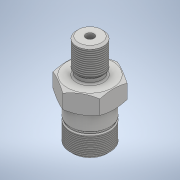
# Autodesk Inventor part: штрундель
Saved by Autodesk Inventor 2021 (Build 250183000, 183)
## iProperties
Created: 2020-04-22
Part Number: штрундель
Material: Типовые
Document SubType Name: Modeling
Designer: 2000
Density: 1 g/cm^3
Appearance: По умолчанию
Mass: 78.5301 g
Surface Area: 176.87 cm^2
Volume: 78.5301 cm^3
Author: 2000
Autodesk Inventor part; units mm, degrees
ref_plane "YZ Plane" through (0, 0, 0) normal (1, 0, 0) x (0, 1, 0)
ref_plane "XZ Plane" through (0, 0, 0) normal (0, 1, 0) x (-1, 0, 0)
ref_plane "XY Plane" through (0, 0, 0) normal (0, 0, 1) x (1, 0, 0)
sketch "Эскиз1" plane through (0, 0, 0) normal (0, 0, 1) x (1, 0, 0)
  line L0 (0, -26.5581) -> (-23, -13.2791)
  line L1 (-23, -13.2791) -> (-23, 13.2791)
  line L2 (-23, 13.2791) -> (0, 26.5581)
  line L3 (0, 26.5581) -> (23, 13.2791)
  line L4 (23, 13.2791) -> (23, -13.2791)
  line L5 (23, -13.2791) -> (0, -26.5581)
  point P0 (0, 0)
  point P1 (0, 0)
  dimension "d127" = 46
  constraints: 12 end point, 1 coincident, 1 vertical, 13 other
  measures "d127" distance between parallel lines of L4 L1
extrude "Выдавливание1" add sketch "Эскиз1" along normal blind 18.8
sketch "Эскиз3" plane through (0, 0, 0) normal (1, 0, 0) x (0, 1, 0)
  line L0 (0, 0) -> (0, 19)
  line L1 (26.5581, 18.8) -> (13.2791, 18.8) projected
  line L2 (13.2791, 0) -> (26.5581, 0) projected
  line L3 (22.25, 18.8) -> (26.5581, 16.3127)
  line L4 (22.25, 0) -> (26.5581, 2.4873)
  line L5 (22.25, 18.8) -> (26.5581, 18.8)
  line L6 (26.5581, 2.4873) -> (26.5581, 0)
  line L7 (26.5581, 0) -> (22.25, 0)
  line L8 (26.5581, 16.3127) -> (26.5581, 18.8)
  dimension "d15" = 30
  dimension "d16" = 30
  dimension "d17" = 44.5
  dimension "d18" = 44.5
  constraints: 14 end point, 3 vertical, 2 collinear, 2 point on line
  measures "d15" angle of L2 L4
  measures "d16" angle of L1 L3
  measures "d17" diameter of L3.start L0
  measures "d18" diameter of L4.start L0
revolve "Вращение2" cut sketch "Эскиз3" angle 360 about axis through (0, 0, 0) along (0, 0, 1)
sketch "Эскиз11" plane through (0, 0, 18.8) normal (0, 0, 1) x (1, 0, 0)
  circle A0 centre (0, 0) radius 11.75
  dimension "d70" = 23.5
  constraints: 1 centre point, 1 coincident
  measures "d70" diameter of A0
extrude "Выдавливание4" add sketch "Эскиз11" along normal blind 5
sketch "Эскиз12" plane through (0, 0, 23.8) normal (0, 0, 1) x (1, 0, 0)
  circle A0 centre (0, 0) radius 13.221
  dimension "d73" = 26.442
  constraints: 1 centre point, 1 coincident
  measures "d73" diameter of A0
extrude "Выдавливание5" add sketch "Эскиз12" along normal blind 27.7
sketch "Эскиз13" plane through (0, 0, 0) normal (0, 0, -1) x (-1, 0, 0)
  circle A0 centre (0, 0) radius 19.5
  dimension "d76" = 39
  constraints: 1 centre point, 1 coincident
  measures "d76" diameter of A0
extrude "Выдавливание6" add sketch "Эскиз13" along normal blind 15.8
sketch "Эскиз14" plane through (0, 0, -15.8) normal (0, 0, -1) x (-1, 0, 0)
  circle A0 centre (0, 0) radius 18.35
  dimension "d79" = 36.7
  constraints: 1 centre point, 1 coincident
  measures "d79" diameter of A0
extrude "Выдавливание7" add sketch "Эскиз14" along normal blind 2.5
sketch "Эскиз16" plane through (0, 0, -18.3) normal (0, 0, -1) x (-1, 0, 0)
  circle A0 centre (0, 0) radius 19.5
  dimension "d82" = 39
  constraints: 1 centre point, 1 coincident
  measures "d82" diameter of A0
extrude "Выдавливание8" add sketch "Эскиз16" along normal blind 21.7
sketch "Эскиз19" plane through (0, 0, 51.5) normal (0, 0, 1) x (1, 0, 0)
  circle A0 centre (0, 0) radius 4
  dimension "d85" = 8
  constraints: 1 centre point, 1 coincident
  measures "d85" diameter of A0
extrude "Выдавливание9" cut sketch "Эскиз19" against normal blind 100
sketch "Эскиз21" plane through (0, 0, -40) normal (0, 0, -1) x (-1, 0, 0)
  circle A0 centre (0, 0) radius 4 projected
  circle A1 centre (0, 0) radius 13
  dimension "d88" = 26
  constraints: 1 centre point, 1 coincident
  measures "d88" diameter of A1
extrude "Выдавливание10" cut sketch "Эскиз21" against normal blind 30
sketch "Эскиз22" plane through (0, 0, -10) normal (0, 0, -1) x (-1, 0, 0)
  point P0 (0, 0)
sketch "Эскиз23" plane through (0, 0, -10) normal (0, 0, -1) x (-1, 0, 0)
  circle A0 centre (0, 0) radius 13.75
  dimension "d91" = 27.5
  constraints: 1 centre point, 1 coincident
  measures "d91" diameter of A0
extrude "Выдавливание11" cut sketch "Эскиз23" along normal blind 9
fillet "Сопряжение1" radius 3 1 edges at (13.75, 0, -10)
thread "Резьба3" size "M26x1.5" class "6H" standard "ANSI Metric M Profile" full length
chamfer "Фаска4" distance 0.75 angle 45 1 edges at (13, 0, -19)
fillet "Сопряжение3" radius 1 2 edges at (13.7499, 0, -19) (13.75, 0, -19)
chamfer "Фаска5" distance 1.6 angle 45 1 edges at (13, 0, -40)
chamfer "Фаска6" distance 3 angle 45 1 edges at (19.5, 0, -40)
thread "Резьба4" size "M39x1.5" class "6g" standard "ANSI Metric M Profile" full length
fillet "Сопряжение4" radius 1 1 edges at (18.35, 0, -15.8)
chamfer "Фаска7" distance 1.15 angle 45 1 edges at (19.5, 0, -18.3)
fillet "Сопряжение5" radius 0.5 2 edges at (18.3501, 0, -18.3) (18.35, 0, -18.3)
thread "Резьба5" size "G26.441x1.814" designation "G 3/4" class "A" standard "DIN Pipe Threads" full length
chamfer "Фаска8" distance 1.471 angle 45 1 edges at (-13.221, 0, 23.8)
fillet "Сопряжение7" radius 0.5 2 edges at (-11.7501, 0, 23.8) (-11.75, 0, 23.8)
fillet "Сопряжение8" radius 1.6 1 edges at (-11.75, 0, 18.8)
chamfer "Фаска9" distance 2 angle 45 1 edges at (-13.221, 0, 51.5)
